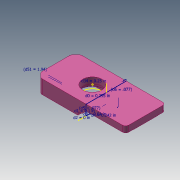
# Autodesk Inventor part: J010513
Saved by Autodesk Inventor 2020.3 (Build 243373000, 373)
## iProperties
RuleStatus: InUse
AfterDocSave0: file://Part Number Cleaner
Created: 2015-03-06
Material: STAINLESS STEEL, 303
Vendor: HHMI: JRC - ID&F
Document SubType Name: Modeling
Designer: ARNOLDJ
Density: 8 g/cm^3
Appearance: Pink
Mass: 3.91869 g
Surface Area: 6.19949 cm^2
Volume: 0.489836 cm^3
Description: MBS WEDGE CLAMP PLATE
Project: COMMON
Part Number: J010513
LAB/DEPT: COMMON
REQUESTING SCIENTIST: COMMON
SURFACE ROUGHNESS: 63 Ra
DESIGN DEPARTMENT: HHMI: JRC - ID&F
SPECIAL FINISH: NONE
ALTERED ITEM PART NUMBER: N/A
ALTERED ITEM VENDOR: N/A
ALTERED ITEM DESCRIPTION: N/A
Revision Number: -
Autodesk Inventor part; units mm, degrees
ref_plane "YZ Plane" through (0, 0, 0) normal (1, 0, 0) x (0, 1, 0)
ref_plane "XZ Plane" through (0, 0, 0) normal (0, 1, 0) x (-1, 0, 0)
ref_plane "XY Plane" through (0, 0, 0) normal (0, 0, 1) x (1, 0, 0)
sketch "Sketch1" plane through (0, 0, 0) normal (1, 0, 0) x (0, 1, 0)
  line L0 (-2.1432, 0) -> (4.5023, 0) projected
  line L1 (0, 7.0231) -> (0, -7.0231) projected
  line L2 (2.54, -5.0165) -> (2.54, 5.0165)
  line L3 (2.54, 5.0165) -> (0, 5.0165)
  line L4 (0, 5.0165) -> (0, -5.0165)
  line L5 (0, -5.0165) -> (2.54, -5.0165)
  line L6 (2.54, -5.0165) -> (0, 5.0165) construction
  line L7 (2.54, 5.0165) -> (0, -5.0165) construction
  line L8 (0, 3.0734) -> (1.016, 3.0734)
  line L9 (1.016, 3.0734) -> (1.016, 5.0165)
  line L10 (0, -3.0734) -> (1.016, -3.0734)
  line L11 (1.016, -3.0734) -> (1.016, -5.0165)
  line L12 (1.27, 0) -> (3.553, 0) construction
  point P0 (0, 0)
  dimension "d0" = 10.033
  dimension "d1" = 2.54
  dimension "d2" = 0
  dimension "d3" = 1.016
  dimension "d4" = 6.1468
  dimension "d5" = 1.9431
  dimension "d6" = 1.9431
  constraints: 22 end point, 6 point on line, 5 perpendicular, 3 parallel, 2 midpoint, 1 horizontal, 1 other
  measures "d0" distance of L2.start L2.end
  measures "d1" distance of L2.end L3.end
  measures "d2" distance from line of point (0, 0) L4
  measures "d3" distance of L8.start L8.end
  measures "d4" distance between parallel lines of L10 L8
  measures "d5" distance of L8.end L9.end
  measures "d6" distance of L10.end L11.end
extrude "Extrusion1" add sketch "Sketch1" along normal blind 9.906 contours L1 L8 L9 L3 L2 L0 | L0 L2 L5 L11 L10 L1
extrude "Extrusion2" add sketch "Sketch1" against normal blind 12.573
sketch "Sketch2" plane through (0, 0, 0) normal (0, 1, 0) x (-1, 0, 0)
  line L0 (-2.3558, 0) -> (14.1351, 0) projected
  line L1 (0, -4.445) -> (0, 4.445) projected
  point P0 (0, 0)
  point P1 (3.429, 0)
  dimension "d11" = 3.429
  constraints: 1 point on line
  measures "d11" distance from line of L1 point (3.429, 0)
hole "Hole1" at (-3.429, 0, 0) direction (0, 1, 0) diameter 4.7625 end through all counterbore diameter 6.223 counterbore depth 1.016
sketch "Sketch3" plane through (9.906, 0, -3.0734) normal (0, -1, 0) x (1, 0, 0)
  line L0 (-22.479, 6.4389) -> (-17.399, 6.4389)
  line L1 (-17.399, 6.4389) -> (-17.399, -0.2921)
  line L2 (-17.399, -0.2921) -> (-22.479, -0.2921)
  line L3 (-22.479, -0.2921) -> (-22.479, 6.4389)
  line L4 (-34.3558, 3.0734) -> (5.726, 3.0734) projected
  line L5 (-9.906, 10.1016) -> (-9.906, -3.9802) projected
  line L6 (-9.906, 3.0734) -> (-28.6298, 3.0734) construction
  line L7 (-22.479, 8.0899) -> (0, 8.0899) projected
  line L8 (-22.479, 6.4389) -> (-11.684, 6.4389)
  line L9 (-11.684, 6.4389) -> (-11.684, 8.0899)
  line L10 (-11.684, 8.0899) -> (-22.479, 8.0899)
  line L11 (-22.479, 8.0899) -> (-22.479, 6.4389)
  line L12 (0, -1.9431) -> (-22.479, -1.9431) projected
  line L13 (-22.479, -0.2921) -> (-11.684, -0.2921)
  line L14 (-11.684, -0.2921) -> (-11.684, -1.9431)
  line L15 (-11.684, -1.9431) -> (-22.479, -1.9431)
  line L16 (-22.479, -1.9431) -> (-22.479, -0.2921)
  dimension "d22" = 5.08
  dimension "d30" = 6.731
  dimension "d45" = 10.795
  dimension "d46" = 10.795
  constraints: 26 end point, 6 parallel, 3 perpendicular, 3 point on line, 2 horizontal, 1 vertical, 1 vertical alignment, 1 other
  measures "d22" distance of L0.end L0.start
  measures "d30" distance of L2.end L0.start
  measures "d45" distance of L0.start L8.end
  measures "d46" distance of L2.end L13.end
extrude "Extrusion3" add sketch "Sketch3" along normal blind 0.889 contours L11 L7 L9 L8 L0 | L0 L1 L4 L3 | L4 L1 L2 L3 | L2 L13 L14 L12 L16
chamfer "Chamfer2" distance 0.254 angle 45 2 edges at (-1.778, -0.889, 4.191) (-1.778, -0.889, -4.191)
fillet "Fillet1" radius 0.7937 2 edges at (9.906, 1.778, 5.0165) (9.906, 1.778, -5.0165)
fillet "Fillet2" [suppressed]
sketch "Sketch4" plane through (0, 0, 0) normal (0, 1, 0) x (-1, 0, 0)
  circle A0 centre (3.429, 0) radius 2.3813 projected
  circle A1 centre (3.429, 0) radius 3.175
  point P0 (0, 0)
  dimension "d34" = 6.35
  constraints: 1 centre point, 1 coincident
  measures "d34" diameter of A1
sketch "Sketch5" plane through (9.906, -0.889, -3.0734) normal (0, -1, 0) x (1, 0, 0)
  line L0 (-26.9748, 3.0734) -> (4.4958, 3.0734) projected
  line L1 (-9.906, 10.0965) -> (-9.906, -3.9497) projected
  line L2 (-22.479, 8.0899) -> (-22.479, -1.9431) projected
  line L3 (-20.955, -0.4191) -> (-22.479, -0.4191)
  line L4 (-22.479, -0.4191) -> (-22.479, 6.5659)
  line L5 (-22.479, 6.5659) -> (-20.955, 6.5659)
  line L6 (-20.955, 6.5659) -> (-20.955, -0.4191)
  line L7 (-20.955, -0.4191) -> (-22.479, 6.5659) construction
  line L8 (-22.479, -0.4191) -> (-20.955, 6.5659) construction
  point P0 (-9.906, 3.0734)
  point P1 (-21.717, 3.0734)
  dimension "d47" = 6.985
  dimension "d48" = 1.524
  constraints: 12 end point, 2 midpoint, 2 parallel, 2 point on line, 1 horizontal, 1 perpendicular
  measures "d47" distance of L5.end L3.start
  measures "d48" distance of L4.end L5.end
extrude "Extrusion4" add sketch "Sketch5" along normal blind 0.3048
chamfer "Chamfer4" distance 1.27 distance2 1.27 1 edges at (-12.573, 0.8255, -5.0165) measured on face at (-12.573, 1.397, 1.1642)
chamfer "Chamfer5" distance 1.27 distance2 1.27 1 edges at (-12.573, 0.8255, 5.0165) measured on face at (-9.0593, 0.254, 5.0165)
fillet "Fillet4" radius 0.7937 2 edges at (-12.573, -1.0414, -3.4925) (-12.573, -1.0414, 3.4925)
fillet "Fillet5" radius 0.7937 4 edges at (-12.573, 0.8255, 3.7465) (-11.303, 0.8255, 5.0165) (-12.573, 0.8255, -3.7465) (-11.303, 0.8255, -5.0165)
fillet "Fillet6" radius 1.651 4 edges at (0, 0.508, -3.0734) (0, 0.508, 3.0734) (-7.493, -0.4445, 3.3655) (-7.493, -0.4445, -3.3655)
sketch "Sketch6" plane through (0, 0, 0) normal (0, 0, 1) x (1, 0, 0)
  line L0 (-11.049, -1.1938) -> (-11.7793, -1.1938) projected
  line L1 (-11.049, -0.889) -> (-11.049, -1.1938) projected
  line L2 (-2.032, -0.889) -> (-10.9742, -0.889) projected
  line L3 (-11.049, -1.1938) -> (-2.032, -0.889)
  point P0 (0, 0)
  dimension "d51" = 1.936
  constraints: 2 end point
  measures "d51" angle of L2 L3
chamfer "Chamfer6" distance 0.9652 angle 45 4 edges at (5.7785, 0, -3.0734) (0, 0, -4.8704) (5.7785, 0, 3.0734) (0, 0, 4.8704) measured on face at (7.1543, 0, 1.0245)
chamfer "Chamfer7" distance 0.9652 angle 45 1 edges at (9.906, 0, 0)
body "Solid1"
